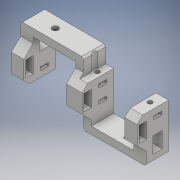
# Autodesk Inventor part: FEMUR
Saved by Autodesk Inventor 2017.3 (Build 213256000, 256)
## iProperties
Created: 2018-01-06
Part Number: FEMUR
Material: Generic
Document SubType Name: Modeling
Designer: Alex
Density: 1 g/cm^3
Appearance: Default
Author: Alex
Autodesk Inventor part; units mm, degrees
ref_plane "YZ Plane" through (0, 0, 0) normal (1, 0, 0) x (0, 1, 0)
ref_plane "XZ Plane" through (0, 0, 0) normal (0, 1, 0) x (-1, 0, 0)
ref_plane "XY Plane" through (0, 0, 0) normal (0, 0, 1) x (1, 0, 0)
sketch "Sketch1" plane through (0, 0, 0) normal (0, 1, 0) x (-1, 0, 0)
  line L0 (34, 17) -> (0, 17)
  line L1 (0, 17) -> (0, -8)
  line L2 (0, -8) -> (34, -8)
  line L3 (34, -8) -> (34, 17)
  line L4 (0, -23.8) -> (0, 23.8) projected
  line L5 (-34, -17) -> (0, -17)
  line L6 (0, -17) -> (0, 8)
  line L7 (0, 8) -> (-34, 8)
  line L8 (-34, 8) -> (-34, -17)
  point P0 (0, 0)
  dimension "d1" = 34
  dimension "d7" = 360
  dimension "d9" = 25
  dimension "d11" = 16
  constraints: 16 end point, 2 parallel, 1 collinear, 1 horizontal, 1 perpendicular, 17 other
  measures "d1" distance of L1.end L2.end
  measures "d9" distance of L2.end L0.start
  measures "d11" distance between parallel lines of L7 L2
extrude "Extrusion1" add sketch "Sketch1" along normal blind 17
sketch "Sketch3" plane through (0, 17, 0) normal (0, 1, 0) x (1, 0, 0)
  line L0 (-27.25, 8) -> (-4.25, 8)
  line L1 (-4.25, 8) -> (-4.25, -13)
  line L2 (-4.25, -13) -> (-27.25, -13)
  line L3 (-27.25, -13) -> (-27.25, 8)
  line L4 (27.25, -8) -> (4.25, -8)
  line L5 (4.25, -8) -> (4.25, 13)
  line L6 (4.25, 13) -> (27.25, 13)
  line L7 (27.25, 13) -> (27.25, -8)
  line L8 (0, 8) -> (-34, 8) projected
  line L9 (-34, -17) -> (0, -17) projected
  line L10 (-34, 8) -> (-34, -17) projected
  line L11 (0, -17) -> (0, -8) projected
  point P0 (0, 0)
  dimension "d16" = 360
  dimension "d20" = 4.25
  dimension "d33" = 4
  dimension "d117" = 23
  constraints: 16 end point, 2 parallel, 1 collinear, 1 horizontal, 1 perpendicular, 17 other
  measures "d20" distance between parallel lines of L11 L1
  measures "d33" distance between parallel lines of L9 L2
  measures "d117" distance of L0.start L0.end
extrude "Extrusion2" cut sketch "Sketch3" against normal blind 12
sketch "Sketch6" plane through (0, 0, -8) normal (0, 0, -1) x (-1, 0, 0)
  circle A0 centre (30, 11) radius 1.25
  circle A1 centre (1.5, 11) radius 1.25
  line L0 (4.25, 5) -> (4.25, 17) projected
  line L1 (27.25, 17) -> (27.25, 5) projected
  point P0 (0, 0)
  point P1 (4.25, 11)
  dimension "d35" = 1.5
  dimension "d36" = 2.5
  dimension "d37" = 1.5
  constraints: 2 centre point, 2 horizontal alignment, 1 equal radius, 1 midpoint
  measures "d35" distance edge to line of A1 L0
  measures "d36" diameter of A1
  measures "d37" distance edge to line of A0 L1
extrude "Extrusion5" cut sketch "Sketch6" against normal blind 10
sketch "Sketch7" plane through (0, 0, 8) normal (0, 0, 1) x (1, 0, 0)
  circle A0 centre (1.5, 11) radius 1.25
  circle A1 centre (30, 11) radius 1.25
  line L0 (27.25, 17) -> (27.25, 5) projected
  line L1 (4.25, 5) -> (4.25, 17) projected
  point P0 (0, 0)
  point P1 (27.25, 11)
  dimension "d40" = 2.5
  dimension "d41" = 1.5
  dimension "d42" = 1.5
  constraints: 2 centre point, 2 horizontal alignment, 1 equal radius, 1 midpoint
  measures "d40" diameter of A1
  measures "d41" distance edge to line of A1 L0
  measures "d42" distance edge to line of A0 L1
extrude "Extrusion6" cut sketch "Sketch7" against normal blind 10
sketch "Sketch8" plane through (34, 0, 8) normal (1, 0, 0) x (0, 0, -1)
  line L0 (21, 17) -> (21, 5) projected
  line L1 (21, 5) -> (0, 5) projected
  line L2 (21, 13.5) -> (12.5, 13.5)
  line L3 (12.5, 13.5) -> (12.5, 8.5)
  line L4 (12.5, 8.5) -> (21, 8.5)
  line L5 (21, 8.5) -> (21, 13.5)
  point P0 (8, 0)
  point P1 (21, 11)
  point P2 (21, 11)
  dimension "d45" = 5
  dimension "d47" = 8.5
  constraints: 8 end point, 2 midpoint, 2 parallel, 1 coincident, 1 collinear, 1 horizontal, 1 perpendicular
  measures "d45" distance of L2.end L3.end
  measures "d47" distance of L3.end L4.end
extrude "Extrusion7" cut sketch "Sketch8" against normal up to surface (6.75 mm away)
sketch "Sketch9" plane through (-34, 0, -8) normal (-1, 0, 0) x (0, 0, 1)
  line L0 (21, 17) -> (21, 5) projected
  line L1 (21, 5) -> (0, 5) projected
  line L2 (21, 8.5) -> (12.5, 8.5)
  line L3 (12.5, 8.5) -> (12.5, 13.5)
  line L4 (12.5, 13.5) -> (21, 13.5)
  line L5 (21, 13.5) -> (21, 8.5)
  point P0 (8, 0)
  point P1 (21, 11)
  point P2 (21, 11)
  dimension "d50" = 5
  dimension "d51" = 8.5
  constraints: 8 end point, 2 midpoint, 2 parallel, 1 coincident, 1 collinear, 1 horizontal, 1 perpendicular
  measures "d50" distance of L2.end L3.end
  measures "d51" distance of L3.end L4.end
extrude "Extrusion8" cut sketch "Sketch9" against normal up to surface (6.75 mm away)
sketch "Sketch10" plane through (0, 0, 0) normal (0, -1, 0) x (1, 0, 0)
  line L0 (34, -17) -> (0, -17) projected
  line L1 (34, 8) -> (34, -17) projected
  line L2 (0, 8) -> (34, 8) projected
  line L3 (0, 17) -> (0, 8) projected
  line L4 (-34, 17) -> (0, 17) projected
  line L5 (-34, -8) -> (-34, 17) projected
  line L6 (0, -8) -> (-34, -8) projected
  line L7 (0, -17) -> (0, -8) projected
  point P0 (0, 0)
extrude "Extrusion9" cut sketch "Sketch10" against normal up to surface (5 mm away)
sketch "Sketch11" plane through (34, 17, -17) normal (0, 0, -1) x (-1, 0, 0)
  circle A0 centre (35.5, -6) radius 1.25 projected
  circle A1 centre (35.5, -6) radius 2.175
  point P0 (34, -17)
  dimension "d56" = 4.35
  constraints: 1 centre point, 1 coincident
  measures "d56" diameter of A1
extrude "Extrusion10" cut sketch "Sketch11" against normal up to surface (9 mm away)
sketch "Sketch12" plane through (-34, 17, 17) normal (0, 0, 1) x (1, 0, 0)
  circle A0 centre (35.5, -6) radius 1.25 projected
  circle A1 centre (35.5, -6) radius 1.25 projected
  circle A2 centre (35.5, -6) radius 2.175
  point P0 (34, -17)
  dimension "d59" = 4.35
  constraints: 1 centre point, 1 coincident
  measures "d59" diameter of A2
extrude "Extrusion11" cut sketch "Sketch12" against normal up to surface (9 mm away)
sketch "Sketch13" plane through (-34, 17, -8) normal (-1, 0, 0) x (0, 0, 1)
  line L0 (3.275, -8.175) -> (5, -8.175)
  line L1 (5, -8.175) -> (5, -3.825)
  line L2 (5, -3.825) -> (3.275, -3.825)
  line L3 (3.275, -3.825) -> (3.275, -8.175)
  line L4 (0, -12) -> (0, 0) projected
  point P0 (8, -17)
  point P1 (3.275, -6)
  point P2 (0, -6)
  dimension "d62" = 5
  dimension "d63" = 1.725
  dimension "d64" = 4.35
  constraints: 8 end point, 2 midpoint, 2 parallel, 1 horizontal, 1 horizontal alignment, 1 perpendicular
  measures "d62" distance between parallel lines of L1 L4
  measures "d63" distance of L0.start L0.end
  measures "d64" distance of L2.end L0.start
extrude "Extrusion12" cut sketch "Sketch13" against normal up to surface (38.25 mm away)
sketch "Sketch14" plane through (34, 17, 8) normal (1, 0, 0) x (0, 0, -1)
  line L0 (5, -8.175) -> (3.275, -8.175)
  line L1 (3.275, -8.175) -> (3.275, -3.825)
  line L2 (3.275, -3.825) -> (5, -3.825)
  line L3 (5, -3.825) -> (5, -8.175)
  line L4 (0, -12) -> (0, 0) projected
  point P0 (8, -17)
  point P1 (3.275, -6)
  point P2 (0, -6)
  dimension "d67" = 5
  dimension "d68" = 4.35
  dimension "d69" = 1.725
  constraints: 8 end point, 2 midpoint, 2 parallel, 1 horizontal, 1 horizontal alignment, 1 perpendicular
  measures "d67" distance between parallel lines of L3 L4
  measures "d68" distance of L0.end L1.end
  measures "d69" distance of L0.start L0.end
extrude "Extrusion13" cut sketch "Sketch14" against normal up to surface (38.25 mm away)
sketch "Sketch15" plane through (4.25, 17, -13) normal (0, 0, 1) x (1, 0, 0)
  circle A0 centre (17, -6) radius 6 construction
  line L0 (0, 0) -> (23, 0) construction
  line L1 (0, -12) -> (23, -12) construction
  line L2 (23, -8.5) -> (23, -12) construction
  line L3 (23, 0) -> (23, -3.5) construction
  line L4 (23, -8.5) -> (23, -3.5) construction
  circle A1 centre (17, -6) radius 1.675
  point P0 (-4.25, -17)
  dimension "d72" = 3.35
  constraints: 3 tangent, 2 centre point, 2 end point, 1 coincident, 1 vertical
  measures "d72" diameter of A1
extrude "Extrusion14" cut sketch "Sketch15" against normal through all
sketch "Sketch16" plane through (-4.25, 17, 13) normal (0, 0, -1) x (-1, 0, 0)
  circle A0 centre (17, -6) radius 6 construction
  line L0 (23, 0) -> (23, -12) construction
  line L1 (0, -12) -> (23, -12) construction
  line L2 (0, 0) -> (23, 0) construction
  circle A1 centre (17, -6) radius 1.675
  point P0 (-4.25, -17)
  dimension "d75" = 3.35
  constraints: 3 tangent, 2 centre point, 1 coincident
  measures "d75" diameter of A1
extrude "Extrusion15" cut sketch "Sketch16" against normal through all
sketch "Sketch17" plane through (-4.25, 17, 13) normal (0, 0, -1) x (-1, 0, 0)
  line L0 (19.925, -3.075) -> (14.075, -3.075)
  line L1 (14.075, -3.075) -> (14.075, -8.925)
  line L2 (14.075, -8.925) -> (19.925, -8.925)
  line L3 (19.925, -8.925) -> (19.925, -3.075)
  circle A0 centre (17, -6) radius 1.675 projected
  point P0 (-4.25, -17)
  point P1 (17, -8.925)
  point P2 (14.075, -6)
  dimension "d78" = 5.85
  constraints: 8 end point, 2 midpoint, 2 parallel, 2 perpendicular, 1 horizontal, 1 horizontal alignment, 1 vertical alignment
  measures "d78" distance of L1.end L2.end
extrude "Extrusion16" cut sketch "Sketch17" against normal blind 2.15
sketch "Sketch18" plane through (4.25, 17, -13) normal (0, 0, 1) x (1, 0, 0)
  line L0 (14.075, -8.925) -> (19.925, -8.925)
  line L1 (19.925, -8.925) -> (19.925, -3.075)
  line L2 (19.925, -3.075) -> (14.075, -3.075)
  line L3 (14.075, -3.075) -> (14.075, -8.925)
  circle A0 centre (17, -6) radius 1.675 projected
  point P0 (-4.25, -17)
  point P1 (17, -3.075)
  point P2 (14.075, -6)
  dimension "d81" = 5.85
  constraints: 8 end point, 2 midpoint, 2 parallel, 2 perpendicular, 1 horizontal, 1 horizontal alignment, 1 vertical alignment
  measures "d81" distance of L1.end L2.end
extrude "Extrusion17" cut sketch "Sketch18" against normal blind 2.15
chamfer "Chamfer1" distance 1 angle 45 4 edges at (-34, 11, 17) (34, 11, -17) (0, 7.2125, 17) (0, 7.2125, -17)
sketch "Sketch21" plane through (4.25, 5, -13) normal (0, -1, 0) x (1, 0, 0)
  line L0 (23, 21) -> (29.75, 21)
  line L1 (29.75, 21) -> (29.75, 5)
  line L2 (29.75, 5) -> (23, 5)
  line L3 (23, 5) -> (23, 21)
  line L4 (-8.5, 21) -> (0, 21)
  line L5 (0, 21) -> (0, 5)
  line L6 (0, 5) -> (-8.5, 5)
  line L7 (-8.5, 5) -> (-8.5, 21)
  line L8 (-38.25, 21) -> (-31.5, 21)
  line L9 (-31.5, 21) -> (-31.5, 5)
  line L10 (-31.5, 5) -> (-38.25, 5)
  line L11 (-38.25, 5) -> (-38.25, 21)
  line L12 (29.75, 21) -> (29.75, -3) projected
  line L13 (23, 0) -> (23, 21) projected
  line L14 (23, 21) -> (29.75, 21) projected
  line L15 (-4.25, 5) -> (-8.5, 5) projected
  line L16 (-4.25, 21) -> (0, 21) projected
  line L17 (0, 21) -> (0, 0) projected
  line L18 (-8.5, 5) -> (-8.5, 26) projected
  line L19 (-31.5, 5) -> (-38.25, 5) projected
  line L20 (-31.5, 26) -> (-31.5, 5) projected
  line L21 (-38.25, 5) -> (-38.25, 29) projected
  point P0 (-4.25, 13)
  constraints: 24 end point, 12 collinear, 6 parallel, 3 horizontal, 3 perpendicular
extrude "Extrusion19" add sketch "Sketch21" along normal blind 5
sketch "Sketch22" plane through (-34, 5, 16) normal (-1, 0, 0) x (0, 0, 1)
  line L0 (-11.75, -4) -> (-20.25, -4)
  line L1 (-20.25, -4) -> (-20.25, 0)
  line L2 (-20.25, 0) -> (-11.75, 0)
  line L3 (-11.75, 0) -> (-11.75, -4)
  line L4 (-8, -5) -> (-24, -5) projected
  line L5 (-8, 0) -> (0, 0) projected
  point P0 (-16, -5)
  point P1 (-16, -4)
  point P2 (-16, -5)
  dimension "d95" = 4
  dimension "d96" = 8.5
  constraints: 8 end point, 2 midpoint, 2 parallel, 1 collinear, 1 horizontal, 1 perpendicular, 1 vertical alignment
  measures "d95" distance of L0.end L1.end
  measures "d96" distance of L0.start L0.end
extrude "Extrusion20" cut sketch "Sketch22" against normal through all
chamfer "Chamfer2" distance 3 angle 45 6 edges at (30.625, 0, 8) (30.625, 0, -8) (0, 0, -8) (0, 0, 8) (-30.625, 0, 8) (-30.625, 0, -8)
chamfer "Chamfer4" distance 2 angle 45 1 edges at (-2.125, 5, 8)
chamfer "Chamfer5" distance 2 angle 45 1 edges at (-30.625, 5, 8)
chamfer "Chamfer6" distance 2 angle 45 1 edges at (2.125, 5, -8)
chamfer "Chamfer7" distance 2 angle 45 1 edges at (30.625, 5, -8)
equation "\"d12\" = servo_B + mat"
equation "\"d21\" = servo_B"
equation "\"d35\" = servo_L"
equation "\"d36\" = servo_H"
equation "\"d37\" = servo_L"
equation "\"d40\" = servo_H"
equation "\"d41\" = servo_L"
equation "\"d42\" = servo_L"
equation "\"d45\" = servo_K"
equation "\"d50\" = servo_K"
equation "\"d63\" = nut_B"
equation "\"d64\" = nut_A"
equation "\"d65\" = 0.5 * servo_A + 0.5 * servo_D + nut_A"
equation "\"d68\" = nut_A"
equation "\"d69\" = nut_B"
equation "\"d70\" = 0.5 * servo_A + 0.5 * servo_D + nut_A"
equation "\"d72\" = screw_m3_A"
equation "\"d75\" = screw_m3_A"
equation "\"d78\" = nut_A_1"
equation "\"d79\" = nut_B_1"
equation "\"d81\" = nut_A_1"
equation "\"d82\" = nut_B_1"
equation "\"mat\" = 5"
equation "\"servo_B\" = 12"
equation "\"servo_L\" = 1.5"
equation "\"servo_H\" = 2.5"
equation "\"servo_K\" = 5"
equation "\"nut_B\" = 1.725"
equation "\"nut_A\" = 4.35"
equation "\"servo_A\" = 23"
equation "\"servo_D\" = 31.5"
equation "\"screw_m3_A\" = 3.35"
equation "\"nut_A_1\" = 5.85"
equation "\"nut_B_1\" = 2.15"
body "Solid1"
